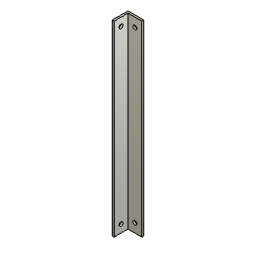
Angle 300 mm Base Side (Autodesk Fusion 360 design; units mm, degrees)
Autodesk Fusion 360 part; units mm, degrees
sketch "Sketch1" plane through (0, 0, 0) normal (0, 1, 0) x (1, 0, 0)
  line L0 (0, -25.4) -> (0, 0)
  line L1 (0, 0) -> (25.4, 0)
  line L2 (12.7, -12.7) -> (11.05, -11.05) construction
  line L3 (3.175, -25.4) -> (3.175, -3.175)
  line L4 (3.175, -3.175) -> (25.4, -3.175)
  line L5 (25.4, -3.175) -> (25.4, 0)
  line L6 (0, -25.4) -> (3.175, -25.4)
  dimension "d1" = 25.4
  dimension "d2" = 25.4
  dimension "d13" = 3.175
  constraint coincident L0.end L2
  constraint coincident L0.end L1.start
  constraint perpendicular L1 L5
  constraint vertical L0
  constraint horizontal L1
  measures "d1" distance of L0.end L1.end
  measures "d2" distance of L0.start L0.end
extrude "Extrude1" add sketch "Sketch1" along normal blind 300
sketch "Sketch2" plane through (3.175, 0, 0) normal (1, 0, 0) x (0, 0, -1)
  line L0 (-25.4, 0) -> (-3.175, 0)
  line L1 (-3.175, 0) -> (-3.175, 300)
  line L2 (-3.175, 300) -> (-25.4, 300)
  line L3 (-25.4, 300) -> (-25.4, 0)
  circle A0 centre (-14.2875, 287.3) radius 2.76
  circle A1 centre (-14.2875, 12.7) radius 2.5546
  line L4 (-14.2875, 300) -> (-14.2875, 0) construction
  dimension "d14" = 12.7
  dimension "d15" = 12.7
  constraint vertical A0.centre A1.centre
  constraint midpoint L2 L4.start
  constraint midpoint L0 L4.end
  constraint coincident A1.centre L4
  measures "d14" distance of L2 A0.centre
  measures "d15" distance of L0 A1.centre
hole "Hole1" at (3.175, 12.7, 14.2875) at (3.175, 287.3, 14.2875) direction (-1, 0, 0) diameter 6.5 end through all
sketch "Sketch3" plane through (0, 0, 3.175) normal (0, 0, 1) x (1, 0, 0)
  line L0 (3.175, 0) -> (25.4, 0)
  line L1 (25.4, 0) -> (25.4, 300)
  line L2 (25.4, 300) -> (3.175, 300)
  line L3 (3.175, 300) -> (3.175, 0)
  line L4 (14.2875, 0) -> (14.2875, 300) construction
  circle A0 centre (14.2875, 285.713) radius 2.8949
  circle A1 centre (14.2875, 14.287) radius 4.0168
  dimension "d19" = 14.287
  dimension "d20" = 14.287
  constraint midpoint L0 L4.start
  constraint midpoint L2 L4.end
  constraint coincident L4 A0.centre
  constraint coincident L4 A1.centre
  measures "d19" distance of L4.end A0.centre
  measures "d20" distance of L4.start A1.centre
hole "Hole2" at (14.2875, 14.287, 3.175) at (14.2875, 285.713, 3.175) direction (0, 0, -1) diameter 6.5 end through all
equation "d14 = ( 25.4 / 2 ) * 1 mm"
equation "d15 = ( 25.4 / 2 ) * 1 mm"
equation "d19 = 25.4 mm - 11.113 mm"
